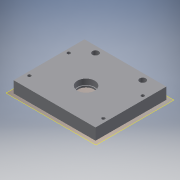
# Autodesk Inventor part: frame bottom
Saved by Autodesk Inventor 2017 (Build 210142000, 142)
## iProperties
Created: 2018-01-19
Part Number: frame bottom
Material: Generic
Document SubType Name: Modeling
Designer: RLanting
Density: 1 g/cm^3
Appearance: Default
Author: RLanting
Autodesk Inventor part; units mm, degrees
ref_plane "YZ Plane" through (0, 0, 0) normal (1, 0, 0) x (0, 1, 0)
ref_plane "XZ Plane" through (0, 0, 0) normal (0, 1, 0) x (-1, 0, 0)
ref_plane "XY Plane" through (0, 0, 0) normal (0, 0, 1) x (1, 0, 0)
ref_plane "Work Plane1" through (0, 0, 0) normal (0, 0, 1) x (1, 0, 0)
sketch "Sketch1" plane through (0, 0, 0) normal (0, 0, 1) x (1, 0, 0)
  circle A0 centre (0, -5) radius 2 projected
  circle A1 centre (94, 45) radius 2 projected
  circle A2 centre (94, -5) radius 2 projected
  circle A3 centre (0, 45) radius 2 projected
  line L0 (5, -10) -> (5, 20) projected
  arc A4 (89, 20) -> (5, 20) centre (47, 20) ccw projected
  line L1 (89, 20) -> (89, -10) projected
  line L2 (99, -20) -> (99, 70) projected
  line L3 (99, 70) -> (-5, 70) projected
  line L4 (-5, 70) -> (-5, -20) projected
  circle A5 centre (47, 20) radius 38
  circle A6 centre (77, 62) radius 4 projected
  circle A7 centre (17, 62) radius 4 projected
  line L5 (89, -10) -> (81, -10) projected
  line L6 (81, -20) -> (81, -10) projected
  line L7 (81, -20) -> (99, -20) projected
  line L8 (-5, -20) -> (13, -20) projected
  line L9 (13, -20) -> (13, -10) projected
  line L10 (5, -10) -> (13, -10) projected
  line L11 (13, -20) -> (81, -20)
  point P0 (0, 0)
  point P1 (5, -20)
  point P2 (89, -20)
  dimension "d0" = 76
  constraints: 2 end point, 1 centre point, 1 coincident, 1 collinear
  measures "d0" diameter of A5
extrude "Extrusion1" add sketch "Sketch1" along normal blind 5.5 contours L10 L9 L8 L4 L3 L2 L7 L6 L5 L1 A4 L0 | L0 A4 L1 L5 L6 L11 L9 L10 | A6 | A7
sketch "Sketch2" plane through (0, 0, 5.5) normal (0, 0, 1) x (1, 0, 0)
  circle A0 centre (47, 20) radius 38 projected
  circle A1 centre (0, 45) radius 2 projected
  circle A2 centre (94, -5) radius 2 projected
  circle A3 centre (94, 45) radius 2 projected
  circle A4 centre (0, -5) radius 2 projected
  line L0 (99, -20) -> (99, 70) projected
  line L1 (99, 70) -> (-5, 70) projected
  line L2 (-5, 70) -> (-5, -20) projected
  circle A5 centre (47, 20) radius 10
  line L3 (-5, -20) -> (99, -20) projected
  point P0 (0, 0)
  dimension "d3" = 20
  constraints: 1 centre point, 1 coincident
  measures "d3" diameter of A5
extrude "Extrusion2" add sketch "Sketch2" along normal blind 2 contours A0 | L3 L2 L1 L0
sketch "Sketch3" plane through (0, 0, 7.5) normal (0, 0, 1) x (1, 0, 0)
  circle A0 centre (47, 20) radius 10 projected
  circle A1 centre (0, -5) radius 2 projected
  circle A2 centre (94, 45) radius 2 projected
  circle A3 centre (94, -5) radius 2 projected
  circle A4 centre (0, 45) radius 2 projected
  line L0 (99, -20) -> (99, 70) projected
  line L1 (99, 70) -> (-5, 70) projected
  line L2 (-5, 70) -> (-5, -20) projected
  circle A5 centre (47, 20) radius 11
  line L3 (-5, -20) -> (99, -20) projected
  point P0 (0, 0)
  dimension "d6" = 22
  constraints: 1 centre point, 1 coincident
  measures "d6" diameter of A5
extrude "Extrusion3" add sketch "Sketch3" along normal blind 7 contours L3 L2 L1 L0
sketch "Sketch4" plane through (0, 0, 0) normal (0, 0, -1) x (-1, 0, 0)
  circle A0 centre (0, -5) radius 2 construction
  circle A1 centre (-94, 45) radius 2 construction
  circle A2 centre (-94, -5) radius 2 construction
  circle A3 centre (0, 45) radius 2 construction
  line L0 (-85, -10) -> (-85, 20) construction
  arc A4 (-9, 20) -> (-85, 20) centre (-47, 20) ccw construction
  line L1 (-9, 20) -> (-9, -10) construction
  line L2 (5, -20) -> (5, 70) construction
  line L3 (5, 70) -> (-99, 70) construction
  line L4 (-99, 70) -> (-99, -20) construction
  line L5 (-77, 62) -> (-17, 62) construction
  circle A5 centre (-77, 62) radius 4
  circle A6 centre (-17, 62) radius 4
  circle A7 centre (-77, 62) radius 4 projected
  circle A8 centre (-17, 62) radius 4 projected
  line L6 (-99, -20) -> (-81, -20) projected
  line L7 (-81, -20) -> (-81, -10) projected
  line L8 (-81, -10) -> (-85, -10) projected
  line L9 (-13, -10) -> (-9, -10) projected
  line L10 (-13, -20) -> (-13, -10) projected
  line L11 (5, -20) -> (-13, -20) projected
  point P0 (0, 0)
  point P1 (-47, 62)
  dimension "d9" = 8
  dimension "d10" = 8
  dimension "d11" = 60
  constraints: 2 centre point, 2 coincident, 2 end point, 1 equal radius, 1 horizontal, 1 midpoint, 1 vertical alignment
  measures "d9" diameter of A5
  measures "d10" distance between parallel lines of L3 L5
  measures "d11" distance of L5.start L5.end
extrude "Extrusion4" cut sketch "Sketch4" against normal through all
body "Solid1"
